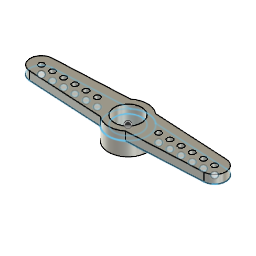
servo (Autodesk Fusion 360 design; units mm, degrees)
part number: 2025-10-09-21-27-08-070
Autodesk Fusion 360 part; units mm, degrees
sketch "Sketch1" plane through (0, 0, 0) normal (0, 0, 1) x (1, 0, 0)
  circle A0 centre (-93.2589, 33.3822) radius 2.4
  line L0 (-91.0241, 36.0759) -> (-77.6483, 35.3351)
  line L1 (-77.6597, 31.3407) -> (-91.0394, 30.6759)
  line L2 (-108.8694, 31.4293) -> (-95.4936, 30.6886)
  line L3 (-95.4783, 36.0886) -> (-108.8581, 35.4238)
  arc A1 (-77.6597, 31.3407) -> (-77.6483, 35.3351) centre (-77.7589, 33.3382) ccw
  arc A2 (-95.4936, 30.6886) -> (-91.0394, 30.6759) centre (-93.2589, 33.3822) ccw
  arc A3 (-91.0241, 36.0759) -> (-95.4783, 36.0886) centre (-93.2589, 33.3822) ccw
  arc A4 (-108.8581, 35.4238) -> (-108.8694, 31.4293) centre (-108.7588, 33.4263) ccw
  circle A5 centre (-108.7588, 33.4263) radius 0.5
  circle A6 centre (-106.7588, 33.4206) radius 0.5
  circle A7 centre (-104.7588, 33.4149) radius 0.5
  circle A8 centre (-102.7588, 33.4092) radius 0.5
  circle A9 centre (-100.7588, 33.4035) radius 0.5
  circle A10 centre (-98.7588, 33.3979) radius 0.5
  line L4 (-93.2589, 33.3822) -> (-93.2296, 43.6849) construction
  circle A11 centre (-87.7589, 33.3666) radius 0.5
  circle A12 centre (-85.7589, 33.3609) radius 0.5
  circle A13 centre (-83.7589, 33.3552) radius 0.5
  circle A14 centre (-81.7589, 33.3496) radius 0.5
  circle A15 centre (-79.7589, 33.3439) radius 0.5
  circle A16 centre (-77.7589, 33.3382) radius 0.5
  circle A17 centre (-93.2589, 33.3822) radius 3.5
  dimension "d1" = 4
  dimension "d2" = 7
  dimension "d3" = 15.5
  dimension "d4" = 4.8
  dimension "d6" = 5.4
  dimension "d10" = 1
  dimension "d11" = 1
  dimension "d12" = 1
  dimension "d13" = 1
  dimension "d14" = 1
  dimension "d15" = 1
  dimension "d16" = 2
  dimension "d17" = 4
  dimension "d18" = 6
  dimension "d19" = 8
  dimension "d20" = 10
  constraint concentric A0 A2
  constraint tangent L1 A1
  constraint tangent L0 A1
  constraint coincident L0.start A2
  constraint concentric A2 A3
  constraint concentric A4 A5
  constraint coincident A0.centre A2.centre
  constraint symmetric A5 L4 A16
  constraint symmetric A6 L4 A15
  constraint symmetric A7 L4 A14
  constraint symmetric A8 L4 A13
  constraint symmetric A9 L4 A12
  constraint symmetric A10 L4 A11
  constraint concentric A3 A17
  measures "d1" diameter of A1
  measures "d2" diameter of A2
  measures "d3" distance of A1.centre A0.centre
  measures "d4" diameter of A0
  measures "d6" distance of L0.start L1.end
  measures "d10" diameter of A5
  measures "d11" diameter of A6
  measures "d12" diameter of A7
  measures "d13" diameter of A8
  measures "d14" diameter of A9
  measures "d15" diameter of A10
  measures "d16" distance of A4.centre A6.centre
  measures "d17" distance of A4.centre A7.centre
  measures "d18" distance of A4.centre A8.centre
  measures "d19" distance of A4.centre A9.centre
  measures "d20" distance of A4.centre A10.centre
extrude "Extrude1" add sketch "Sketch1" along normal blind 1.5
extrude "Extrude2" add sketch "Sketch1" against normal blind 2.5 contours A2 A3 A17
